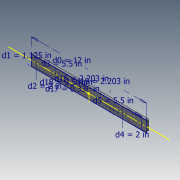
# Autodesk Inventor part: VP TRAY GUIDE CONNECTOR SHELF
Saved by Autodesk Inventor 2018.3 (Build 223284000, 284)
## iProperties
Created: 2019-10-28
Material: Generic
Vendor: HHMI: JRC - ID&F
Document SubType Name: Modeling
Designer: arnoldj
Density: 1 g/cm^3
Appearance: Default
RuleStatus: InUse
AfterDocSave0: file://Part Number Cleaner
DESIGN DEPARTMENT: HHMI: JRC - ID&F
ALTERED ITEM PART NUMBER: N/A
ALTERED ITEM VENDOR: N/A
ALTERED ITEM DESCRIPTION: N/A
Author: arnoldj
Revision Number: 0
Autodesk Inventor part; units mm, degrees
ref_plane "YZ Plane" through (0, 0, 0) normal (1, 0, 0) x (0, 1, 0)
ref_plane "XZ Plane" through (0, 0, 0) normal (0, 1, 0) x (-1, 0, 0)
ref_plane "XY Plane" through (0, 0, 0) normal (0, 0, 1) x (1, 0, 0)
sketch "Sketch1" plane through (0, 0, 0) normal (0, 0, 1) x (1, 0, 0)
  line L0 (0, 20.0025) -> (0, -20.0025) projected
  line L1 (-213.36, 0) -> (213.36, 0) projected
  line L2 (152.4, -14.2875) -> (-152.4, -14.2875)
  line L3 (-152.4, -14.2875) -> (-152.4, 14.2875)
  line L4 (-152.4, 14.2875) -> (152.4, 14.2875)
  line L5 (152.4, 14.2875) -> (152.4, -14.2875)
  line L6 (152.4, -14.2875) -> (-152.4, 14.2875) construction
  line L7 (-152.4, -14.2875) -> (152.4, 14.2875) construction
  line L8 (-65.4562, -5.7531) -> (-55.9562, -5.7531) construction
  line L9 (55.9562, -5.7531) -> (65.4562, -5.7531) construction
  point P0 (0, 0)
  point P1 (-88.9, 0)
  point P2 (-139.7, 0)
  point P3 (88.9, 0)
  point P4 (139.7, 0)
  dimension "d0" = 304.8
  dimension "d1" = 28.575
  dimension "d2" = 50.8
  dimension "d3" = 139.7
  dimension "d4" = 50.8
  dimension "d5" = 139.7
  dimension "d16" = 55.9562
  dimension "d17" = 8.5344
  dimension "d18" = 9.5
  dimension "d19" = 55.9562
  constraints: 16 end point, 4 coincident, 4 point on line, 3 horizontal, 2 midpoint, 2 parallel, 1 collinear, 1 horizontal alignment, 1 perpendicular
  measures "d0" distance of L3.end L4.end
  measures "d1" distance of L2.end L3.end
  measures "d2" distance of point (-88.9, 0) point (-139.7, 0)
  measures "d3" distance from line of L0 point (-139.7, 0)
  measures "d4" distance of point (139.7, 0) point (88.9, 0)
  measures "d5" distance from line of point (139.7, 0) L0
  measures "d16" distance from line of L0 point (-55.956, -5.753)
  measures "d17" distance between parallel lines of L2 L8
  measures "d18" distance of L8.start L8.end
  measures "d19" distance from line of L0 point (55.956, -5.753)
extrude "Extrusion1" add sketch "Sketch1" against normal blind 5.588
hole "Hole1-Tap M4" at (-88.9, 0, 0) at (-139.7, 0, 0) at (88.9, 0, 0) at (139.7, 0, 0) direction (0, 0, -1) diameter 3.1242 depth 25.4 tip angle 118
fillet "Fillet1" radius 3.175 4 edges at (152.4, 14.2875, -2.794) (152.4, -14.2875, -2.794) (-152.4, -14.2875, -2.794) (-152.4, 14.2875, -2.794)
hole "Hole2-Tap M2" at (-65.4562, -5.7531, 0) at (-55.9562, -5.7531, 0) at (55.9562, -5.7531, 0) at (65.4562, -5.7531, 0) direction (0, 0, -1) diameter 1.524 end through all
body "Solid1"
